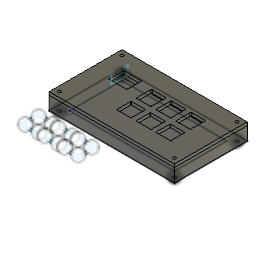
macropad_v1 (Autodesk Fusion 360 design; units mm, degrees)
part number: 2026-06-09-10-43-33-005
Autodesk Fusion 360 part; units mm, degrees
sketch "Sketch1" plane through (0, 0, 0) normal (0, 0, 1) x (1, 0, 0)
  line L0 (0, 0) -> (100.9, 0)
  line L1 (100.9, 0) -> (100.9, 50.4)
  line L2 (100.9, 50.4) -> (0, 50.4)
  line L3 (0, 50.4) -> (0, 0)
  line L4 (-10, 60.4) -> (110.9, 60.4)
  line L5 (110.9, 60.4) -> (110.9, -10)
  line L6 (110.9, -10) -> (-10, -10)
  line L7 (-10, -10) -> (-10, 60.4)
  circle A0 centre (-5, 55.4) radius 1.45
  circle A1 centre (-5, -5) radius 1.45
  circle A2 centre (105.9, 55.4) radius 1.45
  circle A3 centre (105.9, -5) radius 1.45
  dimension "d1" = 100.9
  dimension "d2" = 50.4
  dimension "d3" = 10
  dimension "d4" = 10
  dimension "d5" = 10
  dimension "d6" = 10
  dimension "d7" = 2.9
  dimension "d8" = 2.9
  dimension "d9" = 2.9
  dimension "d10" = 2.9
  dimension "d11" = 5
  dimension "d12" = 5
  dimension "d13" = 5
  dimension "d14" = 5
  dimension "d15" = 5
  dimension "d16" = 5
  dimension "d17" = 5
  dimension "d18" = 5
  constraint horizontal L0
  constraint vertical L1
  constraint horizontal L2
  constraint vertical L3
  constraint coincident L0.start L3.end
  constraint horizontal L4
  constraint vertical L5
  constraint horizontal L6
  constraint vertical L7
  measures "d1" distance of L0.start L0.end
  measures "d2" distance of L0.start L2.end
  measures "d3" distance of L1 L5
  measures "d4" distance of L3 L7
  measures "d5" distance of L2 L4
  measures "d6" distance of L0 L6
  measures "d7" diameter of A0
  measures "d8" diameter of A1
  measures "d9" diameter of A2
  measures "d10" diameter of A3
  measures "d11" distance of L7 A0.centre
  measures "d12" distance of L4 A0.centre
  measures "d13" distance of L6 A1.centre
  measures "d14" distance of L5 A2.centre
  measures "d15" distance of L4 A2.centre
  measures "d16" distance of L6 A3.centre
  measures "d17" distance of L5 A3.centre
  measures "d18" distance of L7 A1.centre
extrude "Extrude1" add sketch "Sketch1" along normal blind 13 makes body 1
extrude "Extrude2" add sketch "Sketch1" along normal blind 3 contours L0 L1 L2 L3 bodies 1
sketch "plate-2026-06-09T01_52_59.866Z" plane through (0, 0, 13) normal (0, 0, 1) x (1, 0, 0)
  line L0 (3.025, -32.525) -> (16.025, -32.525)
  line L1 (3.025, -46.525) -> (16.025, -46.525)
  line L2 (2.525, -33.025) -> (2.525, -46.025)
  line L3 (16.525, -33.025) -> (16.525, -46.025)
  arc A0 (3.025, -32.525) -> (2.525, -33.025) centre (3.025, -33.025) ccw
  arc A1 (16.525, -33.025) -> (16.025, -32.525) centre (16.025, -33.025) ccw
  arc A2 (2.525, -46.025) -> (3.025, -46.525) centre (3.025, -46.025) ccw
  arc A3 (16.025, -46.525) -> (16.525, -46.025) centre (16.025, -46.025) ccw
  line L4 (22.075, -32.525) -> (35.075, -32.525)
  line L5 (22.075, -46.525) -> (35.075, -46.525)
  line L6 (21.575, -33.025) -> (21.575, -46.025)
  line L7 (35.575, -33.025) -> (35.575, -46.025)
  arc A4 (22.075, -32.525) -> (21.575, -33.025) centre (22.075, -33.025) ccw
  arc A5 (35.575, -33.025) -> (35.075, -32.525) centre (35.075, -33.025) ccw
  arc A6 (21.575, -46.025) -> (22.075, -46.525) centre (22.075, -46.025) ccw
  arc A7 (35.075, -46.525) -> (35.575, -46.025) centre (35.075, -46.025) ccw
  line L8 (41.125, -32.525) -> (54.125, -32.525)
  line L9 (41.125, -46.525) -> (54.125, -46.525)
  line L10 (40.625, -33.025) -> (40.625, -46.025)
  line L11 (54.625, -33.025) -> (54.625, -46.025)
  arc A8 (41.125, -32.525) -> (40.625, -33.025) centre (41.125, -33.025) ccw
  arc A9 (54.625, -33.025) -> (54.125, -32.525) centre (54.125, -33.025) ccw
  arc A10 (40.625, -46.025) -> (41.125, -46.525) centre (41.125, -46.025) ccw
  arc A11 (54.125, -46.525) -> (54.625, -46.025) centre (54.125, -46.025) ccw
  line L12 (0, -49.05) -> (57.15, -49.05)
  line L13 (0, -30) -> (57.15, -30)
  line L14 (0, -49.05) -> (0, -30)
  line L15 (57.15, -49.05) -> (57.15, -30)
sketch "Sketch3" plane through (0, 0, 13) normal (0, 0, 1) x (-1, 0, 0)
  circle A0 centre (5, 5) radius 1.45
  circle A1 centre (-105.9, -55.4) radius 1.45
  line L0 (0, 0) -> (0, -50.4)
  line L1 (0, -50.4) -> (-100.9, -50.4)
  line L2 (-100.9, -50.4) -> (-100.9, 0)
  line L3 (-100.9, 0) -> (0, 0)
  circle A2 centre (-105.9, 5) radius 1.45
  circle A3 centre (5, -55.4) radius 1.45
  line L4 (10, 10) -> (-110.9, 10)
  line L5 (-110.9, 10) -> (-110.9, -60.4)
  line L6 (-110.9, -60.4) -> (10, -60.4)
  line L7 (10, -60.4) -> (10, 10)
  line L8 (10, -60.4) -> (-110.9, -60.4)
  line L9 (-110.9, -60.4) -> (-110.9, 10)
  line L10 (-110.9, 10) -> (10, 10)
  line L11 (10, 10) -> (10, -60.4)
  line L12 (-100.9, 0) -> (-100.9, -50.4)
  line L13 (-89.8393, -7.57) -> (-75.8466, -7.5619)
  line L14 (-89.5574, -21.3229) -> (-75.5212, -21.4498)
  line L15 (-89.685, -8.0205) -> (-89.685, -20.6581)
  line L16 (-75.3552, -7.9982) -> (-75.4596, -21.059)
  arc A4 (-89.8393, -7.57) -> (-89.685, -8.0205) centre (-89.9922, -7.874) ccw
  arc A5 (-75.3552, -7.9982) -> (-75.8466, -7.5619) centre (-75.8396, -8.0489) ccw
  arc A6 (-89.685, -20.6581) -> (-89.5574, -21.3229) centre (-89.685, -21.0027) ccw
  arc A7 (-75.5212, -21.4498) -> (-75.4596, -21.059) centre (-75.9243, -21.186) ccw
  line L17 (-70.5258, -7.5339) -> (-56.9206, -7.525)
  line L18 (-70.1538, -21.379) -> (-56.5388, -21.3796)
  line L19 (-70.9171, -7.7251) -> (-70.9171, -20.7393)
  line L20 (-56.425, -7.9587) -> (-56.425, -20.8651)
  arc A8 (-70.5258, -7.5339) -> (-70.9171, -7.7251) centre (-70.5239, -8.0339) ccw
  arc A9 (-56.425, -7.9587) -> (-56.9206, -7.525) centre (-56.9206, -8.025) ccw
  arc A10 (-70.9171, -20.7393) -> (-70.1538, -21.379) centre (-70.5063, -21.0243) ccw
  arc A11 (-56.5388, -21.3796) -> (-56.425, -20.8651) centre (-56.8968, -21.0306) ccw
  line L21 (-51.085, -7.525) -> (-38.085, -7.525)
  line L22 (-51.085, -21.525) -> (-38.085, -21.525)
  line L23 (-51.585, -8.025) -> (-51.585, -21.025)
  line L24 (-37.585, -8.025) -> (-37.585, -21.025)
  arc A12 (-51.085, -7.525) -> (-51.585, -8.025) centre (-51.085, -8.025) ccw
  arc A13 (-37.585, -8.025) -> (-38.085, -7.525) centre (-38.085, -8.025) ccw
  arc A14 (-51.585, -21.025) -> (-51.085, -21.525) centre (-51.085, -21.025) ccw
  arc A15 (-38.085, -21.525) -> (-37.585, -21.025) centre (-38.085, -21.025) ccw
  line L25 (-89.185, -26.5643) -> (-76.1846, -26.5656)
  line L26 (-89.1857, -41.325) -> (-76.1819, -41.325)
  line L27 (-89.7171, -27.0749) -> (-89.7399, -40.094)
  line L28 (-75.6087, -27.0733) -> (-75.5441, -40.1153)
  arc A16 (-89.185, -26.5643) -> (-89.7171, -27.0749) centre (-89.1992, -27.0821) ccw
  arc A17 (-75.6087, -27.0733) -> (-76.1846, -26.5656) centre (-76.1481, -27.1046) ccw
  arc A18 (-89.7399, -40.094) -> (-89.1857, -41.325) centre (-89.0163, -40.5084) ccw
  arc A19 (-76.1819, -41.325) -> (-75.5441, -40.1153) centre (-76.2549, -40.5135) ccw
  line L29 (-70.135, -26.5643) -> (-57.1345, -26.5658)
  line L30 (-70.1351, -41.325) -> (-57.1315, -41.325)
  line L31 (-70.666, -27.0749) -> (-70.6881, -40.0921)
  line L32 (-56.5525, -27.0733) -> (-56.4829, -40.1119)
  arc A20 (-70.135, -26.5643) -> (-70.666, -27.0749) centre (-70.149, -27.0811) ccw
  arc A21 (-56.5525, -27.0733) -> (-57.1345, -26.5658) centre (-57.0939, -27.1067) ccw
  arc A22 (-70.6881, -40.0921) -> (-70.1351, -41.325) centre (-69.9509, -40.5019) ccw
  arc A23 (-57.1315, -41.325) -> (-56.4829, -40.1119) centre (-57.2114, -40.5024) ccw
  line L33 (-51.085, -26.5642) -> (-38.0845, -26.566)
  line L34 (-51.0841, -41.325) -> (-38.081, -41.325)
  line L35 (-51.6155, -27.0749) -> (-51.6373, -40.0893)
  line L36 (-37.4955, -27.0735) -> (-37.4207, -40.1046)
  arc A24 (-51.085, -26.5642) -> (-51.6155, -27.0749) centre (-51.0994, -27.0802) ccw
  arc A25 (-37.4955, -27.0735) -> (-38.0845, -26.566) centre (-38.0381, -27.1077) ccw
  arc A26 (-51.6373, -40.0893) -> (-51.0841, -41.325) centre (-50.8785, -40.4913) ccw
  arc A27 (-38.081, -41.325) -> (-37.4207, -40.1046) centre (-38.1843, -40.4803) ccw
  line L37 (-92.21, -43.85) -> (-35.06, -43.85)
  line L38 (-92.21, -5) -> (-35.06, -5)
  line L39 (-92.21, -43.85) -> (-92.21, -5)
  line L40 (-35.06, -43.85) -> (-35.06, -5)
  line L41 (10, -60.4) -> (-110.9, -60.4)
  line L42 (-110.9, -60.4) -> (-110.9, 10)
  line L43 (-110.9, 10) -> (10, 10)
  line L44 (10, 10) -> (10, -60.4)
  line L45 (-8.2831, -43.484) -> (-25.7831, -43.484)
  line L46 (-25.7831, -43.484) -> (-25.7831, -29.284)
  line L47 (-25.7831, -29.284) -> (-8.2831, -29.284)
  line L48 (-8.2831, -29.284) -> (-8.2831, -43.484)
  dimension "d24" = 6.55
  dimension "d25" = 2.525
  dimension "d26" = 2.525
  dimension "d27" = 2.525
  dimension "d28" = 2.525
  dimension "d29" = 13.0038
  dimension "d30" = 8.69
  dimension "d31" = 2.525
  dimension "d32" = 17.5
  dimension "d33" = 14.2
  dimension "d34" = 9.2769
  constraint horizontal L8
  constraint vertical L9
  constraint horizontal L10
  constraint vertical L11
  constraint coincident L4.end L5.start
  constraint coincident L6.end L7.start
  constraint horizontal L41
  constraint vertical L42
  constraint horizontal L43
  constraint vertical L44
  constraint horizontal L45
  constraint vertical L46
  constraint horizontal L47
  constraint vertical L48
  measures "d24" distance of L1 L37
  measures "d25" distance of L21 L38
  measures "d26" distance of L34 L37
  measures "d27" distance of L30 L37
  measures "d28" distance of L26 L37
  measures "d29" distance of L26.start L26.end
  measures "d30" distance of L12 L39
  measures "d31" distance of L15 L39
  measures "d32" distance of L45.start L45.end
  measures "d33" distance of L45.start L47.end
  measures "d34" distance of L40 L46
extrude "Extrude3" add sketch "Sketch3" along normal blind 3 separate body contours L0 L1 L2 L3 L12 | L4 L5 L6 L7 L8 L9 L10 L11 L41 L42 L43 L44 | L37 L38 L39 L40 makes body 2
sketch "Sketch4" plane through (0, 0, 0) normal (1, 0, 0) x (0, 1, 0)
  line L0 (40, 10) -> (56, 10)
  line L1 (56, 10) -> (56, 2)
  line L2 (56, 2) -> (40, 2)
  line L3 (40, 2) -> (40, 10)
  dimension "d37" = 16
  dimension "d38" = 8
  constraint horizontal L0
  constraint vertical L1
  constraint horizontal L2
  constraint vertical L3
  measures "d37" distance of L0.start L0.end
  measures "d38" distance of L0.start L2.end
sketch "Sketch5" plane through (-10, 0, 0) normal (-1, 0, 0) x (0, -1, 0)
  line L0 (-60.4, 13) -> (10, 13)
  line L1 (10, 13) -> (10, 16)
  line L2 (10, 16) -> (-60.4, 16)
  line L3 (-60.4, 16) -> (-60.4, 13)
  line L4 (-24, 13) -> (-8, 13)
  line L5 (-8, 13) -> (-8, 5)
  line L6 (-8, 5) -> (-24, 5)
  line L7 (-24, 5) -> (-24, 13)
  dimension "d39" = 16
  constraint horizontal L4
  constraint vertical L5
  constraint horizontal L6
  constraint vertical L7
  constraint coincident L0 L4.start
  measures "d39" distance of L4.start L4.end
extrude "Extrude4" cut sketch "Sketch5" against normal blind 10 contours L0 L4 L5 L6 L7 bodies 1
